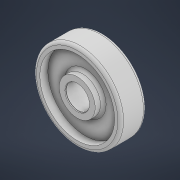
# Autodesk Inventor part: 2
Saved by Autodesk Inventor 2022 (Build 260153000, 153)
## iProperties
Created: 2022-09-05
Part Number: 2
Material: 일반
Document SubType Name: Modeling
Designer: USER
Density: 1 g/cm^3
Appearance: 기본값
Author: USER
Autodesk Inventor part; units mm, degrees
ref_plane "YZ Plane" through (0, 0, 0) normal (1, 0, 0) x (0, 1, 0)
ref_plane "XZ Plane" through (0, 0, 0) normal (0, 1, 0) x (-1, 0, 0)
ref_plane "XY Plane" through (0, 0, 0) normal (0, 0, 1) x (1, 0, 0)
sketch "스케치1" plane through (0, 0, 0) normal (1, 0, 0) x (0, 1, 0)
  line L0 (46, 13.5) -> (0, 13.5)
  line L1 (0, 13.5) -> (0, -13.5)
  line L2 (0, -13.5) -> (46, -13.5)
  line L3 (46, -13.5) -> (46, 13.5)
  line L4 (39.5, 13.5) -> (39.5, 7.7432)
  line L5 (39.5, 5) -> (19, 5)
  line L6 (12.5, 5) -> (12.5, -5)
  line L7 (19, -5) -> (39.5, -5)
  line L8 (46, -5) -> (46, 5)
  line L9 (12.5, 5) -> (12.5, 13.5)
  line L10 (12.5, -5) -> (12.5, -13.5)
  line L11 (19, 13.5) -> (19, 5)
  line L12 (19, -5) -> (19, -13.5)
  line L13 (39.5, 5) -> (39.5, 7.7432)
  line L14 (39.5, -13.5) -> (39.5, -5)
  point P0 (0, 0)
  dimension "d0" = 27
  dimension "d1" = 13.5
  dimension "d2" = 46
  dimension "d3" = 10
  dimension "d4" = 5
  dimension "d5" = 12.5
  dimension "d7" = 39.5
  dimension "d8" = 39.5
  constraints: 30 end point, 8 point on line, 6 perpendicular, 4 parallel, 2 horizontal, 1 collinear, 1 vertical
  measures "d0" distance between parallel lines of L2 L0
  measures "d1" distance from line of L0 point (0, 0)
  measures "d2" distance between parallel lines of L3 L1
  measures "d3" distance between parallel lines of L7 L5
  measures "d4" distance from line of point (0, 0) L5
  measures "d5" distance between parallel lines of L6 L1
  measures "d7" distance between parallel lines of L1 L14
  measures "d8" distance from line of L1 L4.end
revolve "회전1" add sketch "스케치1" angle 360 about axis through (0, 0, 13.5) along (0, 0, -1) contours L3 L2 L14 L7 L12 L10 L6 L9 L0 L11 L5 L13 L4
sketch "스케치2" plane through (0, 0, 13.5) normal (0, 0, 1) x (1, 0, 0)
  circle A0 centre (0, 0) radius 13
  dimension "d10" = 26
  constraints: 1 centre point, 1 coincident
  measures "d10" diameter of A0
extrude "돌출1" cut sketch "스케치2" against normal blind 1
sketch "스케치3" plane through (0, 0, -13.5) normal (0, 0, -1) x (-1, 0, 0)
  circle A0 centre (0, 0) radius 13
  dimension "d13" = 26
  constraints: 1 centre point, 1 coincident
  measures "d13" diameter of A0
extrude "돌출2" cut sketch "스케치3" against normal blind 1
fillet "모깎기1" radius 3 4 edges at (0, -46, 13.5) (0, -46, -13.5) (0, -19, 5) (0, -19, -5)
